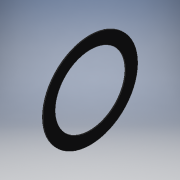
# Autodesk Inventor part: 6007DDU Shield2
Saved by Autodesk Inventor 2019 (Build 230136000, 136)
## iProperties
Created: 2023-07-20
Part Number: 6007DDU Shield2
Material: Generic
Catalog Web Link: www.cadenas.de
Description: contact_sealed_type_dd_ddu_S2-NSK
Vendor: NSK_RB
Document SubType Name: Modeling
Designer: psAdmin
Manufacturer: NSK_RB
Mass: 0.53315 g
Surface Area: 23.5576 cm^2
Volume: 0.53315 cm^3
Density: 1 g/cm^3
Appearance: PSOLRGB-128-128-128
Category: PARTsolutions
Company: NSK_RB
Title: 6007DDU Shield2
Author: Cadenas PARTsolutions
Comments: NSK
PSOL_IDENT_0: {$CADENAS_DATA/23d-libs/nsk_rb/roller_bearings/deep_groove_bb/single_row_dgbb/contact_sealed_type_dd
PSOL_IDENT_1: _ddu_5_s2.prj},195 {VTYP=3D},{NB=6007DDU Shield2},{LINA=6007DDU Shield2},{NN=contact_sealed_type_dd_
PSOL_IDENT_2: ddu_S2},{DATE=15.09.2022 00:32:48},{GEOMDATE=18.05.2018 11:37:52},{VERSION=},{LINEID=1980},{WBVAR=},
PSOL_IDENT_3: {WBNUMERIC=}  {NB=6007DDU Shield2},{LINA=6007DDU Shield2},{KT=DUMMY},{IDNR=21},{STAN=Standard},{ORDE
PSOL_IDENT_4: R=6007DDU},{SD=35},{X=35},{DI1=43.50},{DI2=41.6},{SDE1=54.10},{SDE2=56.00},{D=62},{DD=62},{B=14},{R=
PSOL_IDENT_5: 1.0},{CR1=16000},{COR1=10300},{CR2=1630},{COR2=1050},{FO=14.8},{LG=6700},{A=2.08},{BB=1.90},{DD1=59.
PSOL_IDENT_6: 61},{RO=0.60},{RN=0.5},{DD2=67.7},{F=1.70},{DAM1=40.0},{DA1=41.5},{DA2=57.0},{RA=1.0},{DX=68.5},{CY=
PSOL_IDENT_7: 3.4},{MASS=0.151},{SC=1}
NB: 6007DDU Shield2
NN: contact_sealed_type_dd_ddu_S2
NT: NSK
NBSYN: $ORDER. Shield2
LINA: 6007DDU Shield2
CATALOG: NSK Rolling Bearing
IDNR: 21
STAN: Standard
ORDER: 6007DDU
SD: 35
X: 35
DI1: 43.5
DI2: 41.6
SDE1: 54.1
SDE2: 56
D: 62
DD: 62
B: 14
R: 1
CR1: 16000
COR1: 10300
CR2: 1630
COR2: 1050
FO: 14.8
LG: 6700
A: 2.08
BB: 1.9
DD1: 59.61
RO: 0.6
RN: 0.5
DD2: 67.7
F: 1.7
DAM1: 40
DA1: 41.5
DA2: 57
RA: 1
DX: 68.5
CY: 3.4
MASS: 0.151
SC: 1
SUPPLIER: NSK_RB
ARTICLENO: 6007DDU Shield2
BOMINFO: 6007DDU Shield2
CREATOR: CADENAS GmbH
Autodesk Inventor part; units mm, degrees
ref_plane "YZ Plane" through (0, 0, 0) normal (1, 0, 0) x (0, 1, 0)
ref_plane "XZ Plane" through (0, 0, 0) normal (0, 1, 0) x (-1, 0, 0)
ref_plane "XY Plane" through (0, 0, 0) normal (0, 0, 1) x (1, 0, 0)
sketch "Sketch_1" plane through (0, 0, 0) normal (0, 0, 1) x (1, 0, 0)
  line L0 (0.483, 0) -> (0, 0)
  line L1 (0, 20.8) -> (0.483, 20.8)
  line L2 (0.483, 20.8) -> (0.483, 28)
  line L3 (0.483, 28) -> (0, 28)
  line L4 (0, 28) -> (0, 20.8)
  constraints: 10 end point
revolve "Revolution1" add sketch "Sketch_1" angle 360 about axis through (0.483, 0, 0) along (1, 0, 0)
ref_plane "ip_cst_5_s2_XY" through (0, 0, 0) normal (-1, 0, 0) x (0, 0, -1)
ref_plane "ip_cst_5_s2_YZ" through (0, 0, 0) normal (0, 0, -1) x (0, -1, 0)
ref_plane "ip_cst_5_s2_ZX" through (0, 0, 0) normal (0, -1, 0) x (-1, 0, 0)
body "Solid1"
